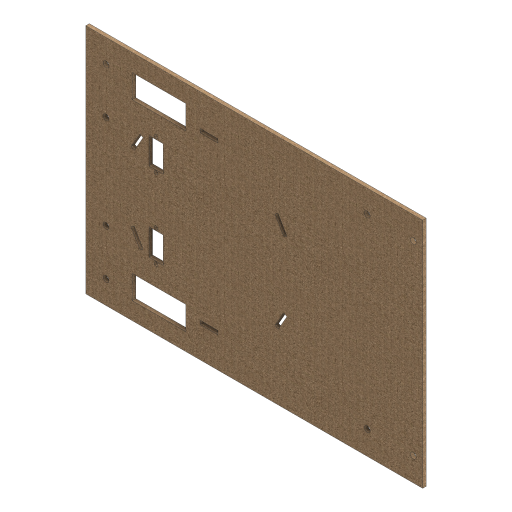
# Autodesk Inventor part: Base_final
Saved by Autodesk Inventor 2024 (Build 280153000, 153)
## iProperties
Created: 2024-04-13
Material: MDF Medium Density Fiberboard
Document SubType Name: Modeling
Designer: 第26組
Density: 0.8 g/cm^3
Appearance: Cardboard - Corrugated
Mass: 132.31 g
Surface Area: 1155.5 cm^2
Volume: 165.387 cm^3
Author: 第26組
Title: Base_final
Autodesk Inventor part; units mm, degrees
ref_plane "YZ Plane" through (0, 0, 0) normal (1, 0, 0) x (0, 1, 0)
ref_plane "XZ Plane" through (0, 0, 0) normal (0, 1, 0) x (-1, 0, 0)
ref_plane "XY Plane" through (0, 0, 0) normal (0, 0, 1) x (1, 0, 0)
sketch "Sketch1" plane through (0, 0, 0) normal (0, 0, 1) x (1, 0, 0)
  line L0 (173.1273, 69.5507) -> (165.6273, 56.5604)
  line L1 (165.6273, 56.5604) -> (163.0292, 58.0604)
  line L2 (163.0292, 58.0604) -> (170.5292, 71.0507)
  line L3 (170.5292, 71.0507) -> (173.1273, 69.5507)
  line L4 (113.6574, 26.5556) -> (98.6574, 26.5556)
  line L5 (98.6574, 26.5556) -> (98.6574, 29.5556)
  line L6 (98.6574, 29.5556) -> (113.6574, 29.5556)
  line L7 (113.6574, 29.5556) -> (113.6574, 26.5556)
  line L8 (46.6875, 142.5507) -> (49.2856, 141.0507)
  line L9 (49.2856, 141.0507) -> (41.7856, 128.0604)
  line L10 (41.7856, 128.0604) -> (39.1875, 129.5604)
  line L11 (39.1875, 129.5604) -> (46.6875, 142.5507)
  line L12 (46.6875, 56.5604) -> (39.1875, 69.5507)
  line L13 (39.1875, 69.5507) -> (41.7856, 71.0507)
  line L14 (41.7856, 71.0507) -> (49.2856, 58.0604)
  line L15 (49.2856, 58.0604) -> (46.6875, 56.5604)
  line L16 (98.6574, 172.5556) -> (113.6574, 172.5556)
  line L17 (113.6574, 172.5556) -> (113.6574, 169.5556)
  line L18 (113.6574, 169.5556) -> (98.6574, 169.5556)
  line L19 (98.6574, 169.5556) -> (98.6574, 172.5556)
  line L20 (165.6273, 142.5507) -> (173.1273, 129.5604)
  line L21 (173.1273, 129.5604) -> (170.5292, 128.0604)
  line L22 (170.5292, 128.0604) -> (163.0292, 141.0507)
  line L23 (163.0292, 141.0507) -> (165.6273, 142.5507)
  line L24 (290, 0) -> (290, 200)
  line L25 (290, 200) -> (0, 200)
  line L26 (0, 200) -> (0, 0)
  line L27 (0, 0) -> (290, 0)
  circle A0 centre (281.9574, 20.463) radius 2.5
  circle A1 centre (49.9574, 20.463) radius 2.5
  circle A2 centre (281.9574, 180.463) radius 2.5
  circle A3 centre (49.9574, 180.463) radius 2.5
  circle A4 centre (242.3574, 20.463) radius 2.5
  circle A5 centre (17.5, 20) radius 2.5
  circle A6 centre (17.5, 180) radius 2.5
  circle A7 centre (242.3574, 180.463) radius 2.5
  line L28 (0, 0) -> (0, 10)
  line L29 (0, 10) -> (0, 15)
  line L30 (0, 200) -> (0, 185)
  line L31 (0, 185) -> (60, 185)
  line L32 (60, 185) -> (60, 175)
  line L33 (60, 175) -> (0, 175)
  line L34 (0, 15) -> (70, 15)
  line L35 (70, 15) -> (70, 25)
  line L36 (70, 25) -> (0, 25)
  line L37 (60, 185) -> (70, 185)
  line L38 (70, 185) -> (70, 175)
  line L39 (70, 175) -> (60, 175)
  line L40 (281.9574, 20.463) -> (242.3574, 20.463)
  line L41 (242.3574, 20.463) -> (130.1488, 20.463)
  circle A8 centre (182.3574, 20.463) radius 2.5
  circle A9 centre (142.7574, 20.463) radius 2.5
  line L42 (0, 100) -> (290, 100)
  line L43 (242.3574, 179.537) -> (130.1488, 179.537)
  circle A10 centre (182.3574, 179.537) radius 2.5
  circle A11 centre (142.7574, 179.537) radius 2.5
  circle A12 centre (17.5, 59.6) radius 2.5
  circle A13 centre (17.5, 140.4) radius 2.5
  line L44 (40, 35.2) -> (86.2, 35.2)
  line L45 (86.2, 35.2) -> (86.2, 15)
  line L46 (86.2, 15) -> (40, 15)
  line L47 (40, 15) -> (40, 35.2)
  line L48 (40, 164.8) -> (86.2, 164.8)
  line L49 (86.2, 164.8) -> (86.2, 185)
  line L50 (86.2, 185) -> (40, 185)
  line L51 (40, 185) -> (40, 164.8)
  line L52 (17.5, 20) -> (17.5, 180)
  line L53 (55, 50) -> (66, 50)
  line L54 (66, 50) -> (66, 82)
  line L55 (66, 82) -> (55, 82)
  line L56 (55, 82) -> (55, 50)
  circle A14 centre (60.5, 52.5) radius 1.5
  circle A15 centre (60.5, 79.5) radius 1.5
  line L57 (54.4, 54.75) -> (66.6, 54.75)
  line L58 (66.6, 54.75) -> (66.6, 77.25)
  line L59 (66.6, 77.25) -> (54.4, 77.25)
  line L60 (54.4, 77.25) -> (54.4, 54.75)
  line L61 (55, 150) -> (66, 150)
  line L62 (66, 150) -> (66, 118)
  line L63 (66, 118) -> (55, 118)
  line L64 (55, 118) -> (55, 150)
  circle A16 centre (60.5, 147.5) radius 1.5
  circle A17 centre (60.5, 120.5) radius 1.5
  line L65 (54.4, 145.25) -> (66.6, 145.25)
  line L66 (66.6, 145.25) -> (66.6, 122.75)
  line L67 (66.6, 122.75) -> (54.4, 122.75)
  line L68 (54.4, 122.75) -> (54.4, 145.25)
  point P0 (66.6, 66)
  point P1 (66, 66)
  point P2 (60.5, 54.75)
  point P3 (60.5, 50)
  point P4 (66.6, 134)
  point P5 (66, 134)
  point P6 (60.5, 145.25)
  point P7 (60.5, 150)
  dimension "d2" = 10
  dimension "d3" = 5
  dimension "d6" = 15
  dimension "d7" = 60
  dimension "d8" = 10
  dimension "d9" = 70
  dimension "d10" = 10
  dimension "d11" = 10
  dimension "d12" = 10
  dimension "d13" = 5
  dimension "d14" = 5
  dimension "d15" = 39.6
  dimension "d16" = 39.6
  dimension "d17" = 60
  dimension "d18" = 8.0426
  dimension "d19" = 39.6
  dimension "d20" = 20.2
  dimension "d21" = 46.2
  dimension "d22" = 15
  dimension "d23" = 40
  dimension "d24" = 17.5
  dimension "d25" = 5
  dimension "d26" = 5
  dimension "d27" = 20
  dimension "d28" = 20
  dimension "d29" = 39.6
  dimension "d30" = 55
  dimension "d31" = 50
  dimension "d32" = 11
  dimension "d33" = 32
  dimension "d34" = 3
  dimension "d35" = 3
  dimension "d36" = 2.5
  dimension "d37" = 2.5
  dimension "d38" = 22.5
  dimension "d39" = 12.2
  constraints: 138 end point, 23 symmetric about line, 18 centre point, 12 point on line, 7 parallel, 7 perpendicular, 6 midpoint, 5 horizontal, 3 vertical alignment, 1 coincident, 1 equal radius, 1 horizontal alignment, 5 other
  measures "d2" distance of L26.end L28.end
  measures "d3" distance of L28.end L29.end
  measures "d6" distance of L25.end L30.end
  measures "d7" distance of L30.end L31.end
  measures "d8" distance of L31.end L32.end
  measures "d9" distance of L29.end L34.end
  measures "d10" distance of L34.end L35.end
  measures "d11" distance of L31.end L37.end
  measures "d12" distance of L37.end L38.end
  measures "d13" diameter of A9
  measures "d14" diameter of A8
  measures "d15" distance of L40.start L40.end
  measures "d16" distance of A9.centre A8.centre
  measures "d17" distance of L40.end A8.centre
  measures "d18" horizontal distance of L24.start L40.start
  measures "d19" distance of L52.start A12.centre
  measures "d20" distance of L44.end L45.end
  measures "d21" distance of L44.start L44.end
  measures "d22" distance between parallel lines of L27 L46
  measures "d23" distance between parallel lines of L26 L47
  measures "d24" horizontal distance of point (0, 0) L52.start
  measures "d25" diameter of A4
  measures "d26" diameter of A0
  measures "d27" vertical distance of point (0, 0) L52.start
  measures "d28" vertical distance of L25.end L52.end
  measures "d29" distance of A13.centre L52.end
  measures "d30" distance between parallel lines of L26 L56
  measures "d31" distance between parallel lines of L27 L53
  measures "d32" distance of L54.end L55.end
  measures "d33" distance of L53.end L54.end
  measures "d34" diameter of A14
  measures "d35" diameter of A15
  measures "d36" vertical distance of L55.end A15.centre
  measures "d37" vertical distance of L53.start A14.centre
  measures "d38" distance of L57.end L58.end
  measures "d39" distance of L57.start L57.end
extrude "Extrusion1" add sketch "Sketch1" along normal blind 3 contours L27 L26 L34 L46 L45 L44 L47 L36 L52 A12 L42 L24 | L42 L52 A13 L33 L51 L48 L49 L50 L37 L31 L26 L25 L24 | L52 A12 L36 L26 L42 | L42 L26 L33 L52 A13 | L26 L36 L47 L34 | L31 L51 L33 L26 | A9 L41 | L41 A9 | A8 L41 | L41 A8 | A11 L43 | L43 A11 | A10 L43 | L43 A10 | L56 L57 L54 L53 | L56 L55 L54 L59 | L61 L62 L65 L64 | L67 L62 L63 L64
body "Solid1"
